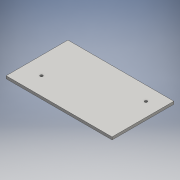
# Autodesk Inventor part: 足フレームの代わり
Saved by Autodesk Inventor 2016 (Build 200138000, 138)
## iProperties
Created: 2018-03-19
Part Number: 足フレームの代わり
Material: 一般
Document SubType Name: Modeling
Designer: Takumi
Appearance: 既定
Surface Area: 179.683 cm^2
Volume: 25.1576 cm^3
Author: Takumi
Autodesk Inventor part; units mm, degrees
ref_plane "YZ Plane" through (0, 0, 0) normal (1, 0, 0) x (0, 1, 0)
ref_plane "XZ Plane" through (0, 0, 0) normal (0, 1, 0) x (-1, 0, 0)
ref_plane "XY Plane" through (0, 0, 0) normal (0, 0, 1) x (1, 0, 0)
sketch "スケッチ1" plane through (0, 0, 0) normal (0, 0, 1) x (1, 0, 0)
  circle A0 centre (0, 0) radius 1.5
  circle A1 centre (84.4097, 34) radius 1.5
  line L0 (-20, 50) -> (100, 50)
  line L1 (100, 50) -> (100, -20)
  line L2 (100, -20) -> (-20, -20)
  line L3 (-20, -20) -> (-20, 50)
  dimension "d0" = 3
  dimension "d1" = 3
  dimension "d2" = 91
  dimension "d3" = 34
  constraints: 8 end point, 2 centre point, 2 parallel, 1 coincident, 1 horizontal, 1 perpendicular
  measures "d0" diameter of A0
  measures "d1" diameter of A1
  measures "d2" distance of point (0, 0) A1.centre
  measures "d3" vertical distance of point (0, 0) A1.centre
extrude "押し出し1" add sketch "スケッチ1" along normal blind 3
